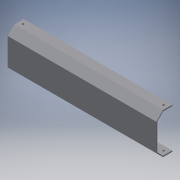
# Autodesk Inventor part: ChassisMainBracket
Saved by Autodesk Inventor 2016 (Build 200138000, 138)
## iProperties
Created: 2015-08-06
Part Number: ChassisMainBracket
Material: Generic
Document SubType Name: Modeling
Designer: lachesis
Density: 1 g/cm^3
Appearance: Default
Author: lachesis
Autodesk Inventor part; units mm, degrees
ref_plane "YZ Plane" through (0, 0, 0) normal (1, 0, 0) x (0, 1, 0)
ref_plane "XZ Plane" through (0, 0, 0) normal (0, 1, 0) x (-1, 0, 0)
ref_plane "XY Plane" through (0, 0, 0) normal (0, 0, 1) x (1, 0, 0)
sketch "Sketch1" plane through (0, 0, 0) normal (1, 0, 0) x (0, 1, 0)
  line L0 (18.8, 0) -> (-18.8, 0)
  line L1 (-18.8, 0) -> (-18.8, 1.6)
  line L2 (-18.8, 1.6) -> (18.8, 1.6)
  line L3 (18.8, 1.6) -> (18.8, 0)
  line L4 (18.8, 1.6) -> (28.2, -7.7473)
  line L5 (28.2, -7.7473) -> (28.2, -20.4563)
  line L6 (28.2, -20.4563) -> (26.6, -20.4563)
  line L7 (26.6, -20.4563) -> (26.6, -7.7563)
  line L8 (26.6, -7.7563) -> (18.8, 0)
  line L9 (0, 0) -> (0, 1.6)
  line L10 (-18.8, 1.6) -> (-28.2, -7.7473)
  line L11 (-28.2, -7.7473) -> (-28.2, -20.4563)
  line L12 (-26.6, -20.4563) -> (-26.6, -7.7563)
  line L13 (-26.6, -7.7563) -> (-18.8, 0)
  line L14 (-28.2, -20.4563) -> (-26.6, -20.4563)
  dimension "d0" = 1.6
  dimension "d1" = 1.6
  dimension "d3" = 11
  dimension "d4" = 12.7
  dimension "d5" = 56.4
  dimension "d8" = 7.8
  constraints: 30 end point, 4 symmetric about line, 3 parallel, 3 perpendicular, 2 horizontal, 2 midpoint, 1 coincident, 1 vertical
  measures "d0" distance between parallel lines of L2 L0
  measures "d1" distance between parallel lines of L7 L5
  measures "d3" distance of L0.start L7.end
  measures "d4" distance of L6.end L7.end
  measures "d5" distance between parallel lines of L11 L5
  measures "d8" horizontal distance of L7.end L0.start
extrude "Extrusion1" add sketch "Sketch1" along normal blind 205.6
sketch "Sketch2" plane through (0, 28.2, -7.7473) normal (0, 1, 0) x (1, 0, 0)
  line L0 (0, 12.709) -> (0, 0) projected
  line L1 (0, 0) -> (205.6, 0) projected
  line L2 (205.6, 12.709) -> (205.6, 0) projected
  line L3 (0, 12.709) -> (205.6, 12.709) projected
  point P0 (0, -7.7473)
  point P1 (5.6, 6.3545)
  point P2 (200, 6.3545)
  point P3 (0, 6.3545)
  point P4 (205.6, 6.3545)
  dimension "d11" = 5.6
  dimension "d12" = 5.6
  constraints: 3 horizontal alignment, 2 midpoint
  measures "d11" distance from line of L0 point (5.6, 6.354)
  measures "d12" distance from line of L2 point (200, 6.354)
hole "Hole1" at (5.6, 28.2, -14.1018) at (200, 28.2, -14.1018) direction (0, -1, 0) diameter 2.459 end up to face face through (68.5333, 26.6, -16.223) facing (0, -1, 0)
sketch "Sketch3" plane through (0, -28.2, -20.4563) normal (0, -1, 0) x (1, 0, 0)
  circle A0 centre (200, 6.3545) radius 1.2295 projected
  circle A1 centre (5.6, 6.3545) radius 1.2295 projected
  point P0 (0, 20.4563)
  constraints: 2 coincident
hole "Hole2" at (200, -28.2, -14.1018) at (5.6, -28.2, -14.1018) direction (0, 1, 0) diameter 2.459 end up to face face through (68.5333, -26.6, -11.9896) facing (0, 1, 0)
equation "\"d12\" = d11"
body "Solid1"
